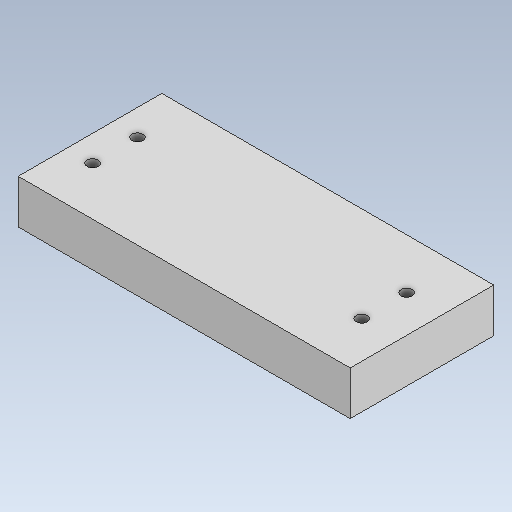
# Autodesk Inventor part: CameraAdapter_part3
Saved by Autodesk Inventor 2020.1 (Build 241239000, 239)
## iProperties
Created: 2019-09-03
Part Number: CameraAdapter_part3
Material: Generic
Document SubType Name: Modeling
Designer: Julian
Density: 1 g/cm^3
Appearance: Default
Author: Julian
Autodesk Inventor part; units mm, degrees
ref_plane "YZ Plane" through (0, 0, 0) normal (1, 0, 0) x (0, 1, 0)
ref_plane "XZ Plane" through (0, 0, 0) normal (0, 1, 0) x (-1, 0, 0)
ref_plane "XY Plane" through (0, 0, 0) normal (0, 0, 1) x (1, 0, 0)
sketch "Sketch1" plane through (0, 0, 0) normal (0, 1, 0) x (-1, 0, 0)
  line L0 (0, 0) -> (150, 0)
  line L1 (150, 0) -> (150, -80)
  line L2 (150, -80) -> (0, -80)
  line L3 (0, -80) -> (0, 0)
  line L4 (150, -80) -> (0, -80)
  line L5 (0, -80) -> (0, -40)
  line L6 (0, -40) -> (150, -40)
  line L7 (150, -40) -> (150, -80)
  line L8 (150, -40) -> (100.4, -40)
  line L9 (100.4, -40) -> (87.7, -40)
  line L10 (87.7, -40) -> (62.3, -40)
  line L11 (62.3, -40) -> (49.6, -40)
  line L12 (0, 0) -> (10.578, 0)
  line L13 (10.578, 0) -> (10.578, -80)
  line L14 (10.578, -80) -> (0, -80)
  line L15 (0, -80) -> (0, 0)
  line L16 (10.578, 0) -> (10.578, -27)
  line L17 (10.578, -27) -> (10.578, -52)
  line L18 (10.578, -52) -> (10.578, -77)
  line L19 (150, 0) -> (160.578, 0)
  line L20 (160.578, 0) -> (160.578, -80)
  line L21 (160.578, -80) -> (150, -80)
  line L22 (150, -80) -> (150, 0)
  line L23 (160.578, 0) -> (160.578, -27)
  line L24 (160.578, -27) -> (160.578, -52)
  line L25 (160.578, -52) -> (160.578, -77)
  line L26 (0, 0) -> (-10, 0)
  line L27 (-10, 0) -> (-10, -80)
  line L28 (-10, -80) -> (0, -80)
  line L29 (0, -80) -> (0, 0)
  line L30 (150, 0) -> (175, 0)
  line L31 (175, 0) -> (175, -80)
  line L32 (175, -80) -> (150, -80)
  line L33 (150, -80) -> (150, 0)
  dimension "d0" = 150
  dimension "d1" = 80
  dimension "d2" = 40
  dimension "d3" = 49.6
  dimension "d4" = 12.7
  dimension "d5" = 25.4
  dimension "d6" = 12.7
  dimension "d34" = 10.578
  dimension "d35" = 27
  dimension "d36" = 25
  dimension "d37" = 25
  dimension "d46" = 27
  dimension "d47" = 25
  dimension "d48" = 25
  dimension "d49" = 10
  dimension "d50" = 25
  dimension "d51" = 14.422
  constraints: 68 end point, 13 point on line, 12 parallel, 6 horizontal, 6 perpendicular, 1 midpoint
  measures "d0" distance of L1.end L2.end
  measures "d1" distance of L0.end L1.end
  measures "d2" distance of L4.end L5.end
  measures "d3" distance of L6.end L8.end
  measures "d4" distance of L8.end L9.end
  measures "d5" distance of L9.end L10.end
  measures "d6" distance of L10.end L11.end
  measures "d34" distance of L13.end L14.end
  measures "d35" distance of L12.end L16.end
  measures "d36" distance of L16.end L17.end
  measures "d37" distance of L17.end L18.end
  measures "d46" distance of L19.end L23.end
  measures "d47" distance of L23.end L24.end
  measures "d48" distance of L24.end L25.end
  measures "d49" distance of L28.end L27.end
  measures "d50" distance of L31.end L32.end
  measures "d51" distance between parallel lines of L24 L31
extrude "Extrusion1" add sketch "Sketch1" along normal blind 24.46
hole "Hole1" at (-49.6, 0, -40) at (-100.4, 0, -40) direction (0, 1, 0) diameter 3.2 depth 4 tip angle 118
hole "Hole2" at (-87.7, 0, -40) at (-62.3, 0, -40) direction (0, 1, 0) diameter 4.917 depth 15 tip angle 118 thread size "M6x1" class "6H" standard "ANSI Metric M Profile"
hole "Hole4" at (-160.578, 0, -27) at (-160.578, 0, -52) at (-10.578, 0, -27) at (-10.578, 0, -52) direction (0, 1, 0) diameter 6.2 end through all counterbore diameter 11 counterbore depth 6 clearance for "Socket Head Cap Screw" size "M6" standard "Ansi Metric M Profile"
body "Solid1"
